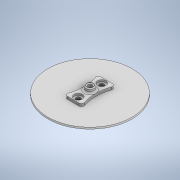
# Autodesk Inventor part: plataforma
Saved by Autodesk Inventor 2022 (Build 260153000, 153)
## iProperties
Created: 2021-12-20
Part Number: plataforma
Material: Genérico
Document SubType Name: Modeling
Designer: JK
Density: 1 g/cm^3
Appearance: Valor por defecto
Author: JK
Autodesk Inventor part; units mm, degrees
ref_plane "YZ Plane" through (0, 0, 0) normal (1, 0, 0) x (0, 1, 0)
ref_plane "XZ Plane" through (0, 0, 0) normal (0, 1, 0) x (-1, 0, 0)
ref_plane "XY Plane" through (0, 0, 0) normal (0, 0, 1) x (1, 0, 0)
sketch "Boceto1" plane through (0, 0, 0) normal (0, 1, 0) x (-1, 0, 0)
  circle A0 centre (0, 0) radius 2.7
  line L0 (10, 20) -> (-10, 20)
  line L1 (-10, 20) -> (-10, -20)
  line L2 (-10, -20) -> (10, -20)
  line L3 (10, -20) -> (10, 20)
  line L4 (10, 20) -> (-10, -20) construction
  line L5 (-10, 20) -> (10, -20) construction
  circle A1 centre (0, 14) radius 2.7
  circle A2 centre (0, -14) radius 2.7
  dimension "d0" = 5.4
  dimension "d1" = 20
  dimension "d2" = 40
  dimension "d3" = 6
  dimension "d4" = 6
  constraints: 12 end point, 3 centre point, 2 equal radius, 2 midpoint, 2 parallel, 1 coincident, 1 horizontal, 1 perpendicular
  measures "d0" diameter of A0
  measures "d1" distance of L1.end L2.end
  measures "d2" distance of L2.end L0.start
  measures "d3" distance from line of L0 A1.centre
  measures "d4" distance from line of L2 A2.centre
extrude "Extrusión1" add sketch "Boceto1" along normal blind 5
sketch "Boceto2" plane through (0, 5, 0) normal (0, 1, 0) x (1, 0, 0)
  circle A0 centre (0, 0) radius 2.7 projected
  circle A1 centre (0, 0) radius 2.7 projected
  circle A2 centre (0, 0) radius 5
  dimension "d21" = 2
  dimension "d22" = 0
  dimension "d7" = 10
  constraints: 1 centre point, 1 coincident
  measures "d7" diameter of A2
extrude "Extrusión2" add sketch "Boceto2" along normal blind 5
sketch "Boceto3" plane through (0, 10, 0) normal (0, 1, 0) x (1, 0, 0)
  circle A0 centre (0, 0) radius 2.575
  circle A1 centre (0, 0) radius 2.7 projected
  dimension "d10" = 5.15
  constraints: 1 centre point, 1 coincident
  measures "d10" diameter of A0
extrude "Extrusión3" add sketch "Boceto3" against normal up to surface (10 mm away)
fillet "Empalme1" radius 3 4 edges at (-10, 2.5, -20) (10, 2.5, -20) (10, 2.5, 20) (-10, 2.5, 20)
fillet "Empalme2" radius 2 1 edges at (-5, 5, 0)
sketch "Boceto4" plane through (0, 5, 0) normal (0, 1, 0) x (1, 0, 0)
  line L0 (10, -17) -> (10, 17) projected
  arc A0 (10, 17) -> (10, -17) centre (56.6667, 0) ccw
  line L1 (10, -17) -> (10, 17) projected
  line L2 (-10, 17) -> (-10, -17) projected
  arc A1 (-7, 20) -> (-10, 17) centre (-7, 17) ccw projected
  arc A2 (-10, -17) -> (-10, 17) centre (-56.6667, 0) ccw
  line L3 (-10, 17) -> (-10, -17) projected
  point P0 (0, 0)
  constraints: 4 point on circle, 2 centre point
extrude "Extrusión4" cut sketch "Boceto4" against normal through all
fillet "Empalme3" radius 3 2 edges at (10, 2.5, 17) (10, 2.5, -17)
fillet "Empalme4" radius 1 2 edges at (-5, 10, 0) (-2.575, 10, 0)
sketch "Boceto5" plane through (0, 5, 0) normal (0, 1, 0) x (1, 0, 0)
  circle A0 centre (0, -14) radius 2.7 projected
  circle A1 centre (0, -14) radius 5
  circle A2 centre (0, 14) radius 2.7 projected
  circle A3 centre (0, 14) radius 5
  point P0 (0, 0)
  dimension "d19" = 10
  dimension "d20" = 10
  constraints: 2 centre point, 2 coincident
  measures "d19" diameter of A1
  measures "d20" diameter of A3
extrude "Extrusión5" cut sketch "Boceto5" against normal blind 2 contours A0 | A1 | A2 | A3
sketch "Boceto7" plane through (0, 0, 0) normal (0, -1, 0) x (1, 0, 0)
  circle A0 centre (0, 0) radius 2.575 projected
  circle A1 centre (0, 0) radius 50
  circle A2 centre (0, -14) radius 2.7 projected
  circle A3 centre (0, 14) radius 2.7 projected
  circle A4 centre (0, 0) radius 2.575 projected
  arc A5 (6.8191, -20) -> (9.6585, -16.0316) centre (6.8191, -17) ccw projected
  arc A6 (9.6585, 16.0316) -> (9.6585, -16.0316) centre (56.6667, 0) ccw projected
  arc A7 (9.6585, 16.0316) -> (6.8191, 20) centre (6.8191, 17) ccw projected
  line L0 (-7, 20) -> (6.8191, 20) projected
  arc A8 (-7, 20) -> (-10, 17) centre (-7, 17) ccw projected
  arc A9 (-10, -17) -> (-10, 17) centre (-56.6667, 0) ccw projected
  arc A10 (-10, -17) -> (-7, -20) centre (-7, -17) ccw projected
  line L1 (6.8191, -20) -> (-7, -20) projected
  dimension "d24" = 100
  constraints: 1 centre point, 1 coincident
  measures "d24" diameter of A1
extrude "Extrusión6" add sketch "Boceto7" against normal blind 2 contours A1
